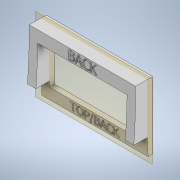
# Autodesk Inventor part: electricalCoverGasket
Saved by Autodesk Inventor 2021.1 (Build 251245000, 245)
## iProperties
Created: 2020-08-29
Part Number: electricalCoverGasket
Material: Generic
Document SubType Name: Modeling
Designer: robst
Density: 1 g/cm^3
Appearance: Default
Author: robst
Autodesk Inventor part; units mm, degrees
ref_plane "YZ Plane" through (0, 0, 0) normal (1, 0, 0) x (0, 1, 0)
ref_plane "XZ Plane" through (0, 0, 0) normal (0, 1, 0) x (-1, 0, 0)
sketch "Sketch1" plane through (0, 0, 0) normal (1, 0, 0) x (0, 1, 0)
  line L0 (0, 0) -> (0, 15.24)
  line L1 (0, 0) -> (-101.6, 0) construction
  arc A0 (-101.6, 0) -> (0, 0) centre (-50.8, 607.4796) ccw
  line L2 (-50.8, -2.1204) -> (-50.8, 0) construction
  line L3 (0, 15.24) -> (101.6, 15.24) construction
  arc A1 (0, 15.24) -> (101.6, 15.24) centre (50.8, 622.7196) ccw
  line L4 (19.05, 0) -> (19.05, 13.947) construction
  line L5 (-19.685, -1.3258) -> (-19.685, -6.4058)
  line L6 (-19.685, -6.4058) -> (57.785, -6.4058)
  line L7 (57.785, -6.4058) -> (57.785, 13.1597)
  dimension "d0" = 15.24
  dimension "d1" = 101.6
  dimension "d3" = 50.8
  dimension "d4" = 2.1204
  dimension "d5" = 609.6
  dimension "d6" = 101.6
  dimension "d7" = 609.6
  dimension "d8" = 19.05
  dimension "d9" = 38.735
  dimension "d10" = 5.08
  dimension "d11" = 77.47
  constraints: 16 end point, 8 point on circle, 3 horizontal, 3 vertical, 2 centre point, 1 midpoint, 1 perpendicular
  measures "d0" distance of L0.start L0.end
  measures "d1" distance of L0.start L1.end
  measures "d3" distance of L2.end L0.start
  measures "d4" distance of L2.start L2.end
  measures "d5" radius of A0
  measures "d6" distance of L0.end L3.end
  measures "d7" radius of A1
  measures "d8" distance between parallel lines of L4 L0
  measures "d9" distance from line of L5 L4.start
  measures "d10" distance of L5.start L5.end
  measures "d11" distance of L5.end L6.end
extrude "Extrusion1" add sketch "Sketch1" along normal mid plane 122.428
sketch "Sketch2" plane through (61.214, 57.785, -6.4058) normal (0, 0, -1) x (-1, 0, 0)
  line L0 (0, -57.785) -> (122.428, -57.785) projected
  line L1 (122.428, -77.47) -> (0, -77.47) projected
  line L2 (122.428, 0) -> (0, 0) projected
  line L3 (61.214, -77.47) -> (61.214, 0) construction
  line L4 (122.428, 0) -> (122.428, -77.47) construction
  line L5 (122.428, -38.735) -> (0, -38.735) construction
  line L6 (0, -77.47) -> (0, 0) construction
  line L7 (112.649, -13.335) -> (9.779, -13.335)
  line L8 (9.779, -13.335) -> (9.779, -64.135)
  line L9 (9.779, -64.135) -> (112.649, -64.135)
  line L10 (112.649, -64.135) -> (112.649, -13.335)
  line L11 (112.649, -13.335) -> (9.779, -64.135) construction
  line L12 (9.779, -13.335) -> (112.649, -64.135) construction
  point P0 (61.214, -57.785)
  point P1 (61.214, -38.735)
  dimension "d14" = 102.87
  dimension "d15" = 50.8
  constraints: 16 end point, 7 midpoint, 2 parallel, 1 perpendicular, 1 vertical
  measures "d14" distance of L7.start L7.end
  measures "d15" distance of L9.end L7.start
extrude "Extrusion2" cut sketch "Sketch2" against normal through all
ref_plane "Work Plane1" through (61.214, 0, 15.24) normal (0, 0, 1) x (1, 0, 0)
sketch "Sketch3" plane through (61.214, 0, 15.24) normal (0, 0, 1) x (1, 0, 0)
  line L0 (-112.649, 44.45) -> (-9.779, 44.45) projected
  line L1 (-122.428, 57.785) -> (0, 57.785) projected
  line L2 (0, 57.785) -> (0, 0) projected
  line L3 (-122.428, 0) -> (-122.428, 57.785) projected
  line L4 (0, -19.685) -> (0, 57.785) construction
  line L5 (0, 51.1175) -> (-122.428, 51.1175) construction
  spline S0 degree 2 poles (-69.9043, 49.158) (-69.9043, 48.4005) (-70.4807, 47.2396) (-70.9582, 46.8608) knots 0 0 0 1 2 2 2
  spline S1 degree 2 poles (-70.9582, 46.8608) (-71.5346, 46.4162) (-72.8437, 46.0375) (-73.8811, 46.0375) knots 0 0 0 1 2 2 2
  line L6 (-73.8811, 46.0375) -> (-76.7957, 46.0375)
  line L7 (-76.7957, 46.0375) -> (-76.7957, 56.1975)
  line L8 (-76.7957, 56.1975) -> (-74.1034, 56.1975)
  spline S2 degree 2 poles (-74.1034, 56.1975) (-73.0166, 56.1975) (-71.9298, 56.0575) (-71.4358, 55.7858) knots 0 0 0 1 2 2 2
  spline S3 degree 2 poles (-71.4358, 55.7858) (-70.8841, 55.4977) (-70.3819, 54.5508) (-70.3819, 53.9086) knots 0 0 0 1 2 2 2
  spline S4 degree 2 poles (-70.3819, 53.9086) (-70.3819, 53.1923) (-71.1393, 52.0561) (-71.8063, 51.735) knots 0 0 0 1 2 2 2
  line L9 (-71.8063, 51.735) -> (-71.8063, 51.6856)
  spline S5 degree 2 poles (-71.8063, 51.6856) (-70.9006, 51.4386) (-69.9043, 50.1295) (-69.9043, 49.158) knots 0 0 0 1 2 2 2
  spline S6 degree 2 poles (-71.3123, 49.1003) (-71.3123, 49.6767) (-71.6416, 50.4177) (-72.1356, 50.6811) knots 0 0 0 1 2 2 2
  spline S7 degree 2 poles (-72.1356, 50.6811) (-72.4567, 50.8458) (-73.2142, 50.9446) (-73.914, 50.9446) knots 0 0 0 1 2 2 2
  line L10 (-73.914, 50.9446) -> (-75.4454, 50.9446)
  line L11 (-75.4454, 50.9446) -> (-75.4454, 47.1902)
  line L12 (-75.4454, 47.1902) -> (-74.3504, 47.1902)
  spline S8 degree 2 poles (-74.3504, 47.1902) (-73.4612, 47.1902) (-72.4402, 47.3548) (-72.045, 47.6183) knots 0 0 0 1 2 2 2
  spline S9 degree 2 poles (-72.045, 47.6183) (-71.6663, 47.89) (-71.3123, 48.5651) (-71.3123, 49.1003) knots 0 0 0 1 2 2 2
  spline S10 degree 2 poles (-71.7898, 53.7193) (-71.7898, 54.0815) (-72.0368, 54.6249) (-72.3085, 54.7814) knots 0 0 0 1 2 2 2
  spline S11 degree 2 poles (-72.3085, 54.7814) (-72.6378, 54.9625) (-73.4365, 55.0448) (-74.1528, 55.0448) knots 0 0 0 1 2 2 2
  line L13 (-74.1528, 55.0448) -> (-75.4454, 55.0448)
  line L14 (-75.4454, 55.0448) -> (-75.4454, 52.0726)
  line L15 (-75.4454, 52.0726) -> (-73.914, 52.0726)
  spline S12 degree 2 poles (-73.914, 52.0726) (-73.28, 52.0726) (-72.679, 52.2043) (-72.3579, 52.4101) knots 0 0 0 1 2 2 2
  spline S13 degree 2 poles (-72.3579, 52.4101) (-72.045, 52.6077) (-71.7898, 53.2417) (-71.7898, 53.7193) knots 0 0 0 1 2 2 2
  line L16 (-69.6573, 46.0375) -> (-66.2323, 56.1975)
  line L17 (-66.2323, 56.1975) -> (-64.5691, 56.1975)
  line L18 (-64.5691, 56.1975) -> (-61.144, 46.0375)
  line L19 (-61.144, 46.0375) -> (-62.5684, 46.0375)
  line L20 (-62.5684, 46.0375) -> (-63.4905, 48.878)
  line L21 (-63.4905, 48.878) -> (-67.3685, 48.878)
  line L22 (-67.3685, 48.878) -> (-68.2906, 46.0375)
  line L23 (-68.2906, 46.0375) -> (-69.6573, 46.0375)
  line L24 (-63.861, 50.0307) -> (-65.4336, 54.8143)
  line L25 (-65.4336, 54.8143) -> (-66.998, 50.0307)
  line L26 (-66.998, 50.0307) -> (-63.861, 50.0307)
  spline S14 degree 2 poles (-56.0805, 45.8564) (-57.0685, 45.8564) (-58.7399, 46.5233) (-59.3491, 47.1902) knots 0 0 0 1 2 2 2
  spline S15 degree 2 poles (-59.3491, 47.1902) (-59.9584, 47.8488) (-60.6253, 49.8249) (-60.6253, 51.1093) knots 0 0 0 1 2 2 2
  spline S16 degree 2 poles (-60.6253, 51.1093) (-60.6253, 52.3854) (-59.9749, 54.2791) (-59.3574, 54.979) knots 0 0 0 1 2 2 2
  spline S17 degree 2 poles (-59.3574, 54.979) (-58.7481, 55.6623) (-57.085, 56.3786) (-56.0558, 56.3786) knots 0 0 0 1 2 2 2
  spline S18 degree 2 poles (-56.0558, 56.3786) (-55.5453, 56.3786) (-54.6479, 56.2304) (-54.2691, 56.1152) knots 0 0 0 1 2 2 2
  spline S19 degree 2 poles (-54.2691, 56.1152) (-53.9398, 56.0081) (-53.2564, 55.7035) (-52.9189, 55.5224) knots 0 0 0 1 2 2 2
  line L27 (-52.9189, 55.5224) -> (-52.9189, 53.8922)
  line L28 (-52.9189, 53.8922) -> (-53.0259, 53.8922)
  spline S20 degree 2 poles (-53.0259, 53.8922) (-53.207, 54.0568) (-53.7669, 54.5179) (-54.1703, 54.7402) knots 0 0 0 1 2 2 2
  spline S21 degree 2 poles (-54.1703, 54.7402) (-54.5573, 54.9543) (-55.4712, 55.226) (-56.064, 55.226) knots 0 0 0 1 2 2 2
  spline S22 degree 2 poles (-56.064, 55.226) (-56.7145, 55.226) (-57.8754, 54.6908) (-58.3117, 54.1803) knots 0 0 0 1 2 2 2
  spline S23 degree 2 poles (-58.3117, 54.1803) (-58.7399, 53.6616) (-59.2174, 52.089) (-59.2174, 51.1093) knots 0 0 0 1 2 2 2
  spline S24 degree 2 poles (-59.2174, 51.1093) (-59.2174, 50.0636) (-58.7152, 48.5569) (-58.2788, 48.0382) knots 0 0 0 1 2 2 2
  spline S25 degree 2 poles (-58.2788, 48.0382) (-57.8507, 47.536) (-56.7062, 47.0255) (-56.064, 47.0255) knots 0 0 0 1 2 2 2
  spline S26 degree 2 poles (-56.064, 47.0255) (-55.4794, 47.0255) (-54.4832, 47.3137) (-54.0962, 47.5277) knots 0 0 0 1 2 2 2
  spline S27 degree 2 poles (-54.0962, 47.5277) (-53.7257, 47.7418) (-53.1741, 48.1864) (-53.0177, 48.3428) knots 0 0 0 1 2 2 2
  line L29 (-53.0177, 48.3428) -> (-52.9189, 48.3428)
  line L30 (-52.9189, 48.3428) -> (-52.9189, 46.7291)
  spline S28 degree 2 poles (-52.9189, 46.7291) (-53.2564, 46.5727) (-53.8492, 46.2845) (-54.2691, 46.1528) knots 0 0 0 1 2 2 2
  spline S29 degree 2 poles (-54.2691, 46.1528) (-54.7137, 46.0046) (-55.4712, 45.8564) (-56.0805, 45.8564) knots 0 0 0 1 2 2 2
  line L31 (-44.2491, 46.0375) -> (-46.0028, 46.0375)
  line L32 (-46.0028, 46.0375) -> (-49.7161, 50.7635)
  line L33 (-49.7161, 50.7635) -> (-50.3089, 50.0966)
  line L34 (-50.3089, 50.0966) -> (-50.3089, 46.0375)
  line L35 (-50.3089, 46.0375) -> (-51.6592, 46.0375)
  line L36 (-51.6592, 46.0375) -> (-51.6592, 56.1975)
  line L37 (-51.6592, 56.1975) -> (-50.3089, 56.1975)
  line L38 (-50.3089, 56.1975) -> (-50.3089, 51.5292)
  line L39 (-50.3089, 51.5292) -> (-46.1428, 56.1975)
  line L40 (-46.1428, 56.1975) -> (-44.4961, 56.1975)
  line L41 (-44.4961, 56.1975) -> (-48.7034, 51.6609)
  line L42 (-48.7034, 51.6609) -> (-44.2491, 46.0375)
  point P0 (-61.214, 0)
  dimension "d18" = 6.6675
  constraints: 2 end point, 2 point on line, 1 horizontal, 1 perpendicular
  measures "d18" distance between parallel lines of L5 L0
emboss "Emboss1" sketch "Sketch3" operation cut depth 2.54 direction (0, 0, 1) wrap yes faces at (-17.145, 53.3401, 13.1249)
sketch "Sketch4" plane through (0, 0, 0) normal (0, 0, 1) x (1, 0, 0)
  line L0 (-61.214, -19.685) -> (61.214, -19.685) projected
  line L1 (51.435, -6.35) -> (-51.435, -6.35) projected
  line L2 (61.214, 0) -> (61.214, -19.685) projected
  line L3 (-61.214, -19.685) -> (-61.214, 0) projected
  line L4 (61.214, -19.685) -> (61.214, 57.785) construction
  line L5 (61.214, -13.0175) -> (-61.214, -13.0175) construction
  line L6 (-61.214, 57.785) -> (-61.214, -19.685) construction
  line L7 (-25.1643, -17.4625) -> (-25.1643, -9.6243)
  line L8 (-25.1643, -9.6243) -> (-28.1469, -9.6243)
  line L9 (-28.1469, -9.6243) -> (-28.1469, -8.5725)
  line L10 (-28.1469, -8.5725) -> (-21.0003, -8.5725)
  line L11 (-21.0003, -8.5725) -> (-21.0003, -9.6243)
  line L12 (-21.0003, -9.6243) -> (-23.9828, -9.6243)
  line L13 (-23.9828, -9.6243) -> (-23.9828, -17.4625)
  line L14 (-23.9828, -17.4625) -> (-25.1643, -17.4625)
  spline S0 degree 2 poles (-13.8033, -9.5883) (-13.299, -10.179) (-12.737, -11.9081) (-12.737, -13.0175) knots 0 0 0 1 2 2 2
  spline S1 degree 2 poles (-12.737, -13.0175) (-12.737, -14.0981) (-13.2846, -15.8488) (-13.8033, -16.4395) knots 0 0 0 1 2 2 2
  spline S2 degree 2 poles (-13.8033, -16.4395) (-14.3508, -17.0591) (-15.7988, -17.6498) (-16.6705, -17.6498) knots 0 0 0 1 2 2 2
  spline S3 degree 2 poles (-16.6705, -17.6498) (-17.5711, -17.6498) (-19.0119, -17.0375) (-19.5378, -16.4395) knots 0 0 0 1 2 2 2
  spline S4 degree 2 poles (-19.5378, -16.4395) (-20.0493, -15.8488) (-20.5968, -14.1125) (-20.5968, -13.0175) knots 0 0 0 1 2 2 2
  spline S5 degree 2 poles (-20.5968, -13.0175) (-20.5968, -11.9008) (-20.0421, -10.2007) (-19.5306, -9.5883) knots 0 0 0 1 2 2 2
  spline S6 degree 2 poles (-19.5306, -9.5883) (-19.0119, -8.9975) (-17.5639, -8.3852) (-16.6705, -8.3852) knots 0 0 0 1 2 2 2
  spline S7 degree 2 poles (-16.6705, -8.3852) (-15.7628, -8.3852) (-14.3076, -9.0192) (-13.8033, -9.5883) knots 0 0 0 1 2 2 2
  spline S8 degree 2 poles (-13.969, -13.0175) (-13.969, -12.1386) (-14.3508, -10.777) (-14.6966, -10.3303) knots 0 0 0 1 2 2 2
  spline S9 degree 2 poles (-14.6966, -10.3303) (-15.0496, -9.8693) (-16.0438, -9.4082) (-16.6633, -9.4082) knots 0 0 0 1 2 2 2
  spline S10 degree 2 poles (-16.6633, -9.4082) (-17.3045, -9.4082) (-18.2699, -9.8549) (-18.6373, -10.3303) knots 0 0 0 1 2 2 2
  spline S11 degree 2 poles (-18.6373, -10.3303) (-18.9903, -10.7842) (-19.3649, -12.153) (-19.3649, -13.0175) knots 0 0 0 1 2 2 2
  spline S12 degree 2 poles (-19.3649, -13.0175) (-19.3649, -14.7681) (-17.8953, -16.6268) (-16.6633, -16.6268) knots 0 0 0 1 2 2 2
  spline S13 degree 2 poles (-16.6633, -16.6268) (-15.4314, -16.6268) (-13.969, -14.7681) (-13.969, -13.0175) knots 0 0 0 1 2 2 2
  spline S14 degree 2 poles (-5.821, -11.2525) (-5.821, -11.8288) (-6.2316, -12.8662) (-6.5991, -13.2264) knots 0 0 0 1 2 2 2
  spline S15 degree 2 poles (-6.5991, -13.2264) (-7.0601, -13.6803) (-8.3065, -14.1486) (-9.2574, -14.1486) knots 0 0 0 1 2 2 2
  line L15 (-9.2574, -14.1486) -> (-10.2588, -14.1486)
  line L16 (-10.2588, -14.1486) -> (-10.2588, -17.4625)
  line L17 (-10.2588, -17.4625) -> (-11.4403, -17.4625)
  line L18 (-11.4403, -17.4625) -> (-11.4403, -8.5725)
  line L19 (-11.4403, -8.5725) -> (-9.207, -8.5725)
  spline S16 degree 2 poles (-9.207, -8.5725) (-8.4145, -8.5725) (-7.3051, -8.8319) (-6.88, -9.1272) knots 0 0 0 1 2 2 2
  spline S17 degree 2 poles (-6.88, -9.1272) (-6.3829, -9.4658) (-5.821, -10.5104) (-5.821, -11.2525) knots 0 0 0 1 2 2 2
  spline S18 degree 2 poles (-7.0529, -11.2885) (-7.0529, -10.8274) (-7.3699, -10.1502) (-7.6941, -9.9341) knots 0 0 0 1 2 2 2
  spline S19 degree 2 poles (-7.6941, -9.9341) (-7.9751, -9.7468) (-8.7243, -9.5955) (-9.279, -9.5955) knots 0 0 0 1 2 2 2
  line L20 (-9.279, -9.5955) -> (-10.2588, -9.5955)
  line L21 (-10.2588, -9.5955) -> (-10.2588, -13.14)
  line L22 (-10.2588, -13.14) -> (-9.4519, -13.14)
  spline S20 degree 2 poles (-9.4519, -13.14) (-8.7315, -13.14) (-7.8454, -12.9094) (-7.5572, -12.6069) knots 0 0 0 1 2 2 2
  spline S21 degree 2 poles (-7.5572, -12.6069) (-7.2907, -12.3403) (-7.0529, -11.7135) (-7.0529, -11.2885) knots 0 0 0 1 2 2 2
  line L23 (-1.2535, -8.1763) -> (-4.7332, -19.3932)
  line L24 (-4.7332, -19.3932) -> (-5.7418, -19.3932)
  line L25 (-5.7418, -19.3932) -> (-2.2765, -8.1763)
  line L26 (-2.2765, -8.1763) -> (-1.2535, -8.1763)
  spline S22 degree 2 poles (6.0083, -14.7321) (6.0083, -15.3949) (5.504, -16.4107) (5.0862, -16.7421) knots 0 0 0 1 2 2 2
  spline S23 degree 2 poles (5.0862, -16.7421) (4.5819, -17.1311) (3.4364, -17.4625) (2.5287, -17.4625) knots 0 0 0 1 2 2 2
  line L27 (2.5287, -17.4625) -> (-0.0216, -17.4625)
  line L28 (-0.0216, -17.4625) -> (-0.0216, -8.5725)
  line L29 (-0.0216, -8.5725) -> (2.3342, -8.5725)
  spline S24 degree 2 poles (2.3342, -8.5725) (3.2851, -8.5725) (4.2361, -8.695) (4.6683, -8.9327) knots 0 0 0 1 2 2 2
  spline S25 degree 2 poles (4.6683, -8.9327) (5.151, -9.1849) (5.5905, -10.0133) (5.5905, -10.5753) knots 0 0 0 1 2 2 2
  spline S26 degree 2 poles (5.5905, -10.5753) (5.5905, -11.202) (4.9277, -12.1962) (4.3441, -12.4772) knots 0 0 0 1 2 2 2
  line L30 (4.3441, -12.4772) -> (4.3441, -12.5204)
  spline S27 degree 2 poles (4.3441, -12.5204) (5.1366, -12.7365) (6.0083, -13.882) (6.0083, -14.7321) knots 0 0 0 1 2 2 2
  spline S28 degree 2 poles (4.7764, -14.7825) (4.7764, -14.2782) (4.4882, -13.6299) (4.056, -13.3993) knots 0 0 0 1 2 2 2
  spline S29 degree 2 poles (4.056, -13.3993) (3.775, -13.2552) (3.1122, -13.1688) (2.4999, -13.1688) knots 0 0 0 1 2 2 2
  line L31 (2.4999, -13.1688) -> (1.1599, -13.1688)
  line L32 (1.1599, -13.1688) -> (1.1599, -16.4539)
  line L33 (1.1599, -16.4539) -> (2.118, -16.4539)
  spline S30 degree 2 poles (2.118, -16.4539) (2.8961, -16.4539) (3.7894, -16.3098) (4.1352, -16.0793) knots 0 0 0 1 2 2 2
  spline S31 degree 2 poles (4.1352, -16.0793) (4.4666, -15.8416) (4.7764, -15.2508) (4.7764, -14.7825) knots 0 0 0 1 2 2 2
  spline S32 degree 2 poles (4.3586, -10.741) (4.3586, -10.424) (4.1424, -9.9485) (3.9047, -9.8116) knots 0 0 0 1 2 2 2
  spline S33 degree 2 poles (3.9047, -9.8116) (3.6165, -9.6531) (2.9177, -9.5811) (2.2909, -9.5811) knots 0 0 0 1 2 2 2
  line L34 (2.2909, -9.5811) -> (1.1599, -9.5811)
  line L35 (1.1599, -9.5811) -> (1.1599, -12.1818)
  line L36 (1.1599, -12.1818) -> (2.4999, -12.1818)
  spline S34 degree 2 poles (2.4999, -12.1818) (3.0546, -12.1818) (3.5805, -12.0665) (3.8615, -11.8864) knots 0 0 0 1 2 2 2
  spline S35 degree 2 poles (3.8615, -11.8864) (4.1352, -11.7135) (4.3586, -11.1588) (4.3586, -10.741) knots 0 0 0 1 2 2 2
  line L37 (6.2244, -17.4625) -> (9.2214, -8.5725)
  line L38 (9.2214, -8.5725) -> (10.6766, -8.5725)
  line L39 (10.6766, -8.5725) -> (13.6736, -17.4625)
  line L40 (13.6736, -17.4625) -> (12.4273, -17.4625)
  line L41 (12.4273, -17.4625) -> (11.6204, -14.977)
  line L42 (11.6204, -14.977) -> (8.2272, -14.977)
  line L43 (8.2272, -14.977) -> (7.4203, -17.4625)
  line L44 (7.4203, -17.4625) -> (6.2244, -17.4625)
  line L45 (11.2962, -13.9685) -> (9.9202, -9.7828)
  line L46 (9.9202, -9.7828) -> (8.5514, -13.9685)
  line L47 (8.5514, -13.9685) -> (11.2962, -13.9685)
  spline S36 degree 2 poles (18.1042, -17.621) (17.2397, -17.621) (15.7772, -17.0375) (15.2441, -16.4539) knots 0 0 0 1 2 2 2
  spline S37 degree 2 poles (15.2441, -16.4539) (14.711, -15.8776) (14.1275, -14.1486) (14.1275, -13.0247) knots 0 0 0 1 2 2 2
  spline S38 degree 2 poles (14.1275, -13.0247) (14.1275, -11.9081) (14.6966, -10.2511) (15.2369, -9.6387) knots 0 0 0 1 2 2 2
  spline S39 degree 2 poles (15.2369, -9.6387) (15.77, -9.0408) (17.2253, -8.414) (18.1258, -8.414) knots 0 0 0 1 2 2 2
  spline S40 degree 2 poles (18.1258, -8.414) (18.5725, -8.414) (19.3577, -8.5437) (19.6891, -8.6445) knots 0 0 0 1 2 2 2
  spline S41 degree 2 poles (19.6891, -8.6445) (19.9773, -8.7382) (20.5752, -9.0048) (20.8706, -9.1632) knots 0 0 0 1 2 2 2
  line L48 (20.8706, -9.1632) -> (20.8706, -10.5897)
  line L49 (20.8706, -10.5897) -> (20.777, -10.5897)
  spline S42 degree 2 poles (20.777, -10.5897) (20.6185, -10.4456) (20.1286, -10.0422) (19.7756, -9.8476) knots 0 0 0 1 2 2 2
  spline S43 degree 2 poles (19.7756, -9.8476) (19.437, -9.6603) (18.6373, -9.4226) (18.1186, -9.4226) knots 0 0 0 1 2 2 2
  spline S44 degree 2 poles (18.1186, -9.4226) (17.5495, -9.4226) (16.5337, -9.8909) (16.1518, -10.3375) knots 0 0 0 1 2 2 2
  spline S45 degree 2 poles (16.1518, -10.3375) (15.7772, -10.7914) (15.3594, -12.1674) (15.3594, -13.0247) knots 0 0 0 1 2 2 2
  spline S46 degree 2 poles (15.3594, -13.0247) (15.3594, -13.9396) (15.7988, -15.258) (16.1807, -15.7119) knots 0 0 0 1 2 2 2
  spline S47 degree 2 poles (16.1807, -15.7119) (16.5553, -16.1513) (17.5567, -16.598) (18.1186, -16.598) knots 0 0 0 1 2 2 2
  spline S48 degree 2 poles (18.1186, -16.598) (18.6301, -16.598) (19.5018, -16.3458) (19.8404, -16.1585) knots 0 0 0 1 2 2 2
  spline S49 degree 2 poles (19.8404, -16.1585) (20.1646, -15.9712) (20.6473, -15.5822) (20.7842, -15.4453) knots 0 0 0 1 2 2 2
  line L50 (20.7842, -15.4453) -> (20.8706, -15.4453)
  line L51 (20.8706, -15.4453) -> (20.8706, -16.8573)
  spline S50 degree 2 poles (20.8706, -16.8573) (20.5752, -16.9942) (20.0565, -17.2464) (19.6891, -17.3616) knots 0 0 0 1 2 2 2
  spline S51 degree 2 poles (19.6891, -17.3616) (19.3001, -17.4913) (18.6373, -17.621) (18.1042, -17.621) knots 0 0 0 1 2 2 2
  line L52 (28.4566, -17.4625) -> (26.9221, -17.4625)
  line L53 (26.9221, -17.4625) -> (23.673, -13.3273)
  line L54 (23.673, -13.3273) -> (23.1543, -13.9108)
  line L55 (23.1543, -13.9108) -> (23.1543, -17.4625)
  line L56 (23.1543, -17.4625) -> (21.9729, -17.4625)
  line L57 (21.9729, -17.4625) -> (21.9729, -8.5725)
  line L58 (21.9729, -8.5725) -> (23.1543, -8.5725)
  line L59 (23.1543, -8.5725) -> (23.1543, -12.6573)
  line L60 (23.1543, -12.6573) -> (26.7997, -8.5725)
  line L61 (26.7997, -8.5725) -> (28.2405, -8.5725)
  line L62 (28.2405, -8.5725) -> (24.5592, -12.542)
  line L63 (24.5592, -12.542) -> (28.4566, -17.4625)
  point P0 (0, 0)
  dimension "d21" = 6.6675
  constraints: 2 end point, 2 point on line, 1 horizontal, 1 perpendicular
  measures "d21" distance between parallel lines of L5 L0
emboss "Emboss2" sketch "Sketch4" operation cut depth 2.54 direction (0, 0, 1) wrap yes faces at (-17.145, -15.238, -1.0822)
equation "\"d0\" = sidingDepth"
equation "\"d1\" = sidingHeight"
equation "\"d5\" = radiusOfCurvature"
equation "\"d6\" = sidingHeight"
equation "\"d7\" = radiusOfCurvature"
equation "\"d8\" = 0.5 * electricalPlugHeight"
equation "\"d9\" = 0.5 * coverHeight"
equation "\"d10\" = partDepth"
equation "\"d11\" = coverHeight"
equation "\"d12\" = coverWidth"
equation "\"d14\" = insideHoleWidth"
equation "\"d15\" = insideHoleHeight"
equation "\"sidingHeight\" = 101.6"
equation "\"sidingDepth\" = 15.24"
equation "\"radiusOfCurvature\" = 609.6"
equation "\"partDepth\" = 5.08"
equation "\"coverHeight\" = 77.47"
equation "\"coverWidth\" = 122.428"
equation "\"electricalPlugHeight\" = 38.1"
equation "\"insideHoleWidth\" = 102.87"
equation "\"insideHoleHeight\" = 50.8"
body "Solid1"
